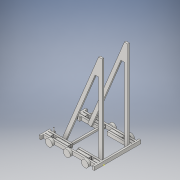
# Autodesk Inventor part: base
Saved by Autodesk Inventor 2016 (Build 200138000, 138)
## iProperties
Created: 2018-01-19
Part Number: base
Material: Generic
Document SubType Name: Modeling
Designer: New User
Density: 1 g/cm^3
Appearance: Default
Author: New User
Autodesk Inventor part; units mm, degrees
ref_plane "YZ Plane" through (0, 0, 0) normal (1, 0, 0) x (0, 1, 0)
ref_plane "XZ Plane" through (0, 0, 0) normal (0, 1, 0) x (-1, 0, 0)
ref_plane "XY Plane" through (0, 0, 0) normal (0, 0, 1) x (1, 0, 0)
sketch "Sketch1" plane through (0, 0, 0) normal (0, 1, 0) x (-1, 0, 0)
  line L0 (0, -685.8) -> (0, 0)
  line L1 (25.4, -38.1) -> (689.3542, -38.1)
  line L2 (787.4, -63.5) -> (25.4, -63.5)
  line L3 (787.4, -647.7) -> (25.4, -647.7)
  line L4 (787.4, -622.3) -> (25.4, -622.3)
  line L5 (787.4, -114.3) -> (457.2, -114.3)
  line L6 (457.2, -114.3) -> (457.2, -139.7)
  line L7 (457.2, -546.1) -> (457.2, -571.5)
  line L8 (457.2, -571.5) -> (787.4, -571.5)
  line L9 (25.4, -571.5) -> (355.6, -571.5)
  line L10 (355.6, -571.5) -> (355.6, -546.1)
  line L11 (355.6, -546.1) -> (25.4, -546.1)
  line L12 (25.4, -139.7) -> (355.6, -139.7)
  line L13 (355.6, -114.3) -> (25.4, -114.3)
  line L14 (355.6, -114.3) -> (355.6, -139.7)
  line L15 (0, 0) -> (25.4, 0)
  line L16 (787.4, 0) -> (812.8, 0)
  line L17 (787.4, -63.5) -> (787.4, -114.3)
  line L18 (787.4, -571.5) -> (787.4, -622.3)
  line L19 (787.4, -647.7) -> (787.4, -685.8)
  line L20 (812.8, -685.8) -> (787.4, -685.8)
  line L21 (25.4, -685.8) -> (0, -685.8)
  line L22 (25.4, -647.7) -> (25.4, -685.8)
  line L23 (25.4, -571.5) -> (25.4, -622.3)
  line L24 (25.4, -139.7) -> (25.4, -546.1)
  line L25 (25.4, 0) -> (25.4, -38.1)
  line L26 (25.4, -63.5) -> (25.4, -114.3)
  line L27 (689.3542, -38.1) -> (787.4, -38.1)
  line L28 (787.4, -38.1) -> (787.4, 0)
  line L29 (812.8, -152.4) -> (787.4, -152.4)
  line L30 (787.4, -533.4) -> (812.8, -533.4)
  line L31 (812.8, 0) -> (812.8, -152.4)
  line L32 (812.8, -533.4) -> (812.8, -685.8)
  line L33 (787.4, -139.7) -> (787.4, -152.4)
  line L34 (508, -139.7) -> (508, -546.1)
  line L35 (482.6, -139.7) -> (482.6, -546.1)
  line L36 (457.2, -139.7) -> (482.6, -139.7)
  line L37 (508, -139.7) -> (787.4, -139.7)
  line L38 (660.4, -546.1) -> (508, -546.1)
  line L39 (482.6, -546.1) -> (457.2, -546.1)
  line L40 (660.4, -546.1) -> (787.4, -546.1)
  line L41 (787.4, -546.1) -> (787.4, -533.4)
  dimension "d0" = 685.8
  dimension "d1" = 812.8
  dimension "d4" = 25.4
  dimension "d5" = 25.4
  dimension "d8" = 50.8
  dimension "d9" = 25.4
  dimension "d10" = 50.8
  dimension "d42" = 330.2
  dimension "d43" = 25.4
  dimension "d44" = 25.4
  dimension "d45" = 25.4
  dimension "d46" = 25.4
  dimension "d47" = 330.2
  dimension "d54" = 152.4
  dimension "d55" = 152.4
  dimension "d56" = 25.4
  dimension "d57" = 304.8
  constraints: 84 end point, 74 perpendicular, 7 horizontal, 6 parallel, 4 point on line, 3 equal length
  measures "d0" distance of L16.end L20.start
  measures "d1" distance of L20.start L0.start
  measures "d4" distance between parallel lines of L3 L4
  measures "d5" distance between parallel lines of L2 L1
  measures "d8" distance between parallel lines of L4 L9
  measures "d9" distance of L9.end L10.end
  measures "d10" distance between parallel lines of L2 L5
  measures "d42" distance between parallel lines of L10 L23
  measures "d43" distance between parallel lines of L23 L0
  measures "d44" distance between parallel lines of L0 L24
  measures "d45" distance between parallel lines of L0 L26
  measures "d46" distance between parallel lines of L0 L25
  measures "d47" distance of L7.end L8.end
  measures "d54" distance between parallel lines of L20 L30
  measures "d55" distance between parallel lines of L16 L29
  measures "d56" distance between parallel lines of L35 L34
  measures "d57" distance between parallel lines of L34 L31
extrude "Extrusion1" add sketch "Sketch1" along normal blind 50.8
sketch "Sketch2" plane through (-689.3542, 0, -38.1) normal (0, 0, 1) x (1, 0, 0)
  circle A0 centre (16.2542, 17.78) radius 50.8
  circle A1 centre (282.9542, 17.78) radius 50.8
  circle A2 centre (549.6542, 17.78) radius 50.8
  line L0 (-98.0458, 0) -> (-98.0458, 50.8) projected
  line L1 (663.9542, 0) -> (663.9542, 50.8) projected
  line L2 (-98.0458, 0) -> (663.9542, 0) projected
  point P0 (689.3542, 0)
  dimension "d13" = 101.6
  dimension "d14" = 114.3
  dimension "d15" = 114.3
  dimension "d16" = 381
  dimension "d17" = 17.78
  dimension "d18" = 17.78
  dimension "d19" = 17.78
  constraints: 3 centre point, 2 equal radius
  measures "d13" diameter of A0
  measures "d14" distance from line of L0 A0.centre
  measures "d15" distance from line of L1 A2.centre
  measures "d16" distance from line of L0 A1.centre
  measures "d17" distance from line of L2 A0.centre
  measures "d18" distance from line of L2 A1.centre
  measures "d19" distance from line of L2 A2.centre
extrude "Extrusion2" add sketch "Sketch2" along normal blind 38.1
sketch "Sketch3" plane through (-25.4, 0, -647.7) normal (0, 0, -1) x (-1, 0, 0)
  arc A0 (152.9047, 50.8) -> (75.6953, 50.8) centre (114.3, 17.78) ccw projected
  circle A1 centre (114.3, 17.78) radius 50.8
  arc A2 (419.6047, 50.8) -> (342.3953, 50.8) centre (381, 17.78) ccw projected
  circle A3 centre (381, 17.78) radius 50.8
  arc A4 (686.3047, 50.8) -> (609.0953, 50.8) centre (647.7, 17.78) ccw projected
  circle A5 centre (647.7, 17.78) radius 50.8
  point P0 (-25.4, 0)
  constraints: 3 centre point, 3 coincident
extrude "Extrusion3" add sketch "Sketch3" along normal blind 38.1
sketch "Sketch4" plane through (-25.4, 0, -63.5) normal (-1, 0, 0) x (0, 0, 1)
  line L0 (-50.8, 50.8) -> (0, 50.8) projected
  line L1 (0, 0) -> (-50.8, 0) projected
  line L2 (-6.35, 50.8) -> (-44.45, 50.8)
  line L3 (-50.8, 44.45) -> (-50.8, 6.35)
  line L4 (-44.45, 0) -> (-6.35, 0)
  line L5 (0, 6.35) -> (0, 44.45)
  arc A0 (-44.45, 50.8) -> (-50.8, 44.45) centre (-44.45, 44.45) ccw
  arc A1 (-50.8, 6.35) -> (-44.45, 0) centre (-44.45, 6.35) ccw
  arc A2 (0, 44.45) -> (-6.35, 50.8) centre (-6.35, 44.45) ccw
  arc A3 (-6.35, 0) -> (0, 6.35) centre (-6.35, 6.35) ccw
  line L6 (-558.8, 50.8) -> (-508, 50.8) projected
  line L7 (-508, 0) -> (-508, 50.8) projected
  line L8 (-552.45, 50.8) -> (-514.35, 50.8)
  line L9 (-508, 44.45) -> (-508, 6.35)
  line L10 (-514.35, 0) -> (-552.45, 0)
  line L11 (-558.8, 6.35) -> (-558.8, 44.45)
  arc A4 (-508, 44.45) -> (-514.35, 50.8) centre (-514.35, 44.45) ccw
  arc A5 (-558.8, 6.35) -> (-552.45, 0) centre (-552.45, 6.35) ccw
  arc A6 (-552.45, 50.8) -> (-558.8, 44.45) centre (-552.45, 44.45) ccw
  arc A7 (-514.35, 0) -> (-508, 6.35) centre (-514.35, 6.35) ccw
  line L12 (-552.45, 3.175) -> (-514.35, 3.175)
  arc A8 (-514.35, 3.175) -> (-511.175, 6.35) centre (-514.35, 6.35) ccw
  line L13 (-511.175, 6.35) -> (-511.175, 44.45)
  arc A9 (-511.175, 44.45) -> (-514.35, 47.625) centre (-514.35, 44.45) ccw
  line L14 (-514.35, 47.625) -> (-552.45, 47.625)
  arc A10 (-552.45, 47.625) -> (-555.625, 44.45) centre (-552.45, 44.45) ccw
  line L15 (-555.625, 44.45) -> (-555.625, 6.35)
  arc A11 (-555.625, 6.35) -> (-552.45, 3.175) centre (-552.45, 6.35) ccw
  line L16 (-6.35, 3.175) -> (-44.45, 3.175)
  arc A12 (-47.625, 6.35) -> (-44.45, 3.175) centre (-44.45, 6.35) ccw
  line L17 (-47.625, 6.35) -> (-47.625, 44.45)
  arc A13 (-44.45, 47.625) -> (-47.625, 44.45) centre (-44.45, 44.45) ccw
  line L18 (-44.45, 47.625) -> (-6.35, 47.625)
  arc A14 (-3.175, 44.45) -> (-6.35, 47.625) centre (-6.35, 44.45) ccw
  line L19 (-3.175, 44.45) -> (-3.175, 6.35)
  arc A15 (-6.35, 3.175) -> (-3.175, 6.35) centre (-6.35, 6.35) ccw
  point P0 (63.5, 0)
  dimension "d24" = 6.35
  dimension "d25" = 6.35
  constraints: 32 end point, 32 point on circle, 16 centre point, 16 tangent, 8 parallel, 8 point on line, 6 equal radius, 4 perpendicular, 2 horizontal, 14 other
  measures "d24" radius of A0
  measures "d25" radius of A4
extrude "Extrusion4" add sketch "Sketch4" along normal blind 762 contours L0 A2 L5 A3 L1 A1 L3 A0 | L6 A4 L7 A7 L10 A5 L11 A6
sketch "Sketch5" plane through (0, 50.8, 0) normal (0, 1, 0) x (1, 0, 0)
  line L0 (-25.4, 63.5) -> (-787.4, 63.5) projected
  line L1 (-355.6, 114.3) -> (-25.4, 114.3) projected
  line L2 (-101.6, 63.5) -> (-152.4, 63.5)
  line L3 (-152.4, 63.5) -> (-152.4, 114.3)
  line L4 (-152.4, 114.3) -> (-101.6, 114.3)
  line L5 (-101.6, 114.3) -> (-101.6, 63.5)
  line L6 (-355.6, 114.3) -> (-457.2, 114.3) projected
  line L7 (-342.9, 63.5) -> (-457.2, 63.5)
  line L8 (-457.2, 63.5) -> (-457.2, 114.3)
  line L9 (-457.2, 114.3) -> (-342.9, 114.3)
  line L10 (-342.9, 114.3) -> (-342.9, 63.5)
  line L11 (-787.4, 114.3) -> (-457.2, 114.3) projected
  line L12 (-647.7, 63.5) -> (-711.2, 63.5)
  line L13 (-711.2, 63.5) -> (-711.2, 114.3)
  line L14 (-711.2, 114.3) -> (-647.7, 114.3)
  line L15 (-647.7, 114.3) -> (-647.7, 63.5)
  line L16 (-457.2, 571.5) -> (-787.4, 571.5) projected
  line L17 (-25.4, 622.3) -> (-787.4, 622.3) projected
  line L18 (-711.2, 571.5) -> (-647.7, 571.5)
  line L19 (-647.7, 571.5) -> (-647.7, 622.3)
  line L20 (-647.7, 622.3) -> (-711.2, 622.3)
  line L21 (-711.2, 622.3) -> (-711.2, 571.5)
  line L22 (-355.6, 571.5) -> (-457.2, 571.5) projected
  line L23 (-457.2, 571.5) -> (-355.6, 571.5)
  line L24 (-355.6, 571.5) -> (-355.6, 622.3)
  line L25 (-355.6, 622.3) -> (-457.2, 622.3)
  line L26 (-457.2, 622.3) -> (-457.2, 571.5)
  line L27 (-25.4, 571.5) -> (-355.6, 571.5) projected
  line L28 (-165.1, 622.3) -> (-101.6, 622.3)
  line L29 (-101.6, 622.3) -> (-101.6, 571.5)
  line L30 (-101.6, 571.5) -> (-165.1, 571.5)
  line L31 (-165.1, 571.5) -> (-165.1, 622.3)
  line L32 (-25.4, 546.1) -> (-25.4, 139.7) projected
  line L33 (-787.4, 139.7) -> (-787.4, 152.4) projected
  point P0 (0, 0)
  point P1 (-787.4, 546.1)
  dimension "d28" = 63.5
  dimension "d29" = 50.8
  dimension "d30" = 76.2
  dimension "d31" = 76.2
  dimension "d32" = 63.5
  dimension "d33" = 63.5
  dimension "d34" = 76.2
  dimension "d35" = 190.5
  dimension "d36" = 190.5
  dimension "d37" = 190.5
  dimension "d38" = 190.5
  constraints: 48 end point, 13 point on line, 12 parallel, 6 horizontal, 6 perpendicular
  measures "d28" distance of L29.end L30.end
  measures "d29" distance of L3.end L4.end
  measures "d30" distance between parallel lines of L32 L29
  measures "d31" distance between parallel lines of L32 L5
  measures "d32" distance between parallel lines of L21 L19
  measures "d33" distance between parallel lines of L13 L15
  measures "d34" distance between parallel lines of L33 L21
  measures "d35" distance between parallel lines of L19 L26
  measures "d36" distance between parallel lines of L8 L15
  measures "d37" distance between parallel lines of L24 L31
  measures "d38" distance between parallel lines of L10 L3
extrude "Extrusion5" cut sketch "Sketch5" against normal blind 50.8 contours L0 L3 L1 L5 | L0 L8 L6 L1 L10 | L0 L13 L11 L15 | L26 L17 L24 L22 | L16 L21 L17 L19 | L31 L17 L29 L27
sketch "Sketch7" plane through (-25.4, 0, -139.7) normal (0, 0, -1) x (-1, 0, 0)
  point P0 (-25.4, 0)
sketch "Sketch8" plane through (0, 50.8, 0) normal (0, 1, 0) x (1, 0, 0)
  line L0 (-508, 139.7) -> (-787.4, 139.7) projected
  line L1 (-508, 139.7) -> (-482.6, 139.7)
  line L2 (-482.6, 139.7) -> (-482.6, 546.1)
  line L3 (-482.6, 546.1) -> (-508, 546.1)
  line L4 (-508, 546.1) -> (-508, 139.7)
  point P0 (0, 0)
  constraints: 8 end point, 2 parallel, 1 horizontal, 1 perpendicular
extrude "Extrusion7" cut sketch "Sketch8" against normal blind 25.4
sketch "Sketch9" plane through (-25.4, 0, -139.7) normal (0, 0, -1) x (-1, 0, 0)
  line L0 (330.2, 0) -> (0, 0) projected
  line L1 (0, 0) -> (50.8, 0)
  line L2 (50.8, 0) -> (50.8, 993.775)
  line L3 (50.8, 1346.2) -> (0, 1346.2)
  line L4 (0, 1346.2) -> (0, 0)
  line L5 (609.0953, 50.8) -> (419.6047, 50.8) projected
  line L6 (50.8, 1346.2) -> (584.2, 50.8)
  line L7 (584.2, 50.8) -> (537.2264, 31.4579)
  line L8 (537.2264, 31.4579) -> (101.7518, 1089.0389)
  line L9 (50.8, 1089.0389) -> (101.7518, 1089.0389)
  line L10 (50.8, 993.775) -> (50.8, 1089.0389)
  point P0 (-25.4, 0)
  dimension "d61" = 1346.2
  dimension "d67" = 50.8
  dimension "d68" = 50.8
  constraints: 18 end point, 3 parallel, 3 perpendicular, 2 horizontal, 1 point on line
  measures "d61" distance of L3.end L0.end
  measures "d67" distance between parallel lines of L6 L8
  measures "d68" distance between parallel lines of L4 L2
extrude "Extrusion8" add sketch "Sketch9" along normal blind 25.4
sketch "Sketch10" plane through (-355.6, 0, -546.1) normal (0, 0, 1) x (1, 0, 0)
  line L0 (-431.8, 0) -> (330.2, 0) projected
  line L1 (330.2, 0) -> (279.4, 0)
  line L2 (279.4, 1346.2) -> (330.2, 1346.2)
  line L3 (330.2, 1346.2) -> (330.2, 0)
  line L4 (279.4, 1346.2) -> (-260.35, 31.75)
  line L5 (-260.35, 31.75) -> (-213.3576, 12.4536)
  line L6 (-213.3576, 12.4536) -> (166.1331, 936.625)
  line L7 (279.4, 909.6375) -> (279.4, 0)
  line L8 (330.2, 50.8) -> (254.5047, 50.8) projected
  line L9 (279.4, 1089.0389) -> (228.7185, 1089.0389)
  line L10 (166.1331, 936.625) -> (228.7185, 1089.0389)
  line L11 (279.4, 909.6375) -> (279.4, 1089.0389)
  line L12 (279.4, 50.8) -> (279.4, 1089.0389) projected
  point P0 (355.6, 0)
  point P1 (279.4, 1212.7791)
  constraints: 20 end point, 2 horizontal, 2 parallel, 1 collinear, 1 perpendicular, 1 vertical
extrude "Extrusion9" add sketch "Sketch10" along normal blind 25.4
sketch "Sketch11" plane through (-787.4, 0, -546.1) normal (0, 0, 1) x (1, 0, 0)
  line L0 (25.4, 0) -> (50.8, 0)
  line L1 (50.8, 0) -> (50.8, 50.8)
  line L2 (50.8, 50.8) -> (25.4, 50.8)
  line L3 (25.4, 50.8) -> (25.4, 0)
  line L4 (0, 0) -> (0, 50.8) projected
  point P0 (787.4, 0)
  dimension "d75" = 25.4
  dimension "d76" = 50.8
  dimension "d77" = 25.4
  constraints: 8 end point, 2 parallel, 1 horizontal, 1 perpendicular
  measures "d75" distance of L1.end L2.end
  measures "d76" distance of L2.end L0.start
  measures "d77" distance between parallel lines of L3 L4
extrude "Extrusion10" add sketch "Sketch11" along normal blind 25.4
sketch "Sketch12" plane through (-508, 0, -139.7) normal (0, 0, -1) x (-1, 0, 0)
  line L0 (203.2, 0) -> (279.4, 0) projected
  line L1 (254, 0) -> (228.6, 0)
  line L2 (228.6, 0) -> (228.6, 50.8)
  line L3 (228.6, 50.8) -> (254, 50.8)
  line L4 (254, 50.8) -> (254, 0)
  line L5 (279.4, 0) -> (279.4, 50.8) projected
  point P0 (-508, 0)
  dimension "d80" = 25.4
  dimension "d81" = 25.4
  constraints: 8 end point, 2 parallel, 1 horizontal, 1 perpendicular, 1 point on line
  measures "d80" distance of L2.end L3.end
  measures "d81" distance between parallel lines of L5 L4
extrude "Extrusion11" add sketch "Sketch12" along normal blind 25.4
sketch "Sketch13" plane through (0, 50.8, 0) normal (0, 1, 0) x (1, 0, 0)
  circle A0 centre (-749.3, 533.4) radius 6.35
  circle A1 centre (-749.3, 152.4) radius 6.35
  line L0 (-736.6, 520.7) -> (-762, 520.7) projected
  line L1 (-736.6, 546.1) -> (-736.6, 520.7) projected
  line L2 (-736.6, 139.7) -> (-736.6, 165.1) projected
  line L3 (-736.6, 165.1) -> (-762, 165.1) projected
  point P0 (0, 0)
  dimension "d84" = 12.7
  dimension "d85" = 12.7
  dimension "d86" = 12.7
  dimension "d87" = 12.7
  dimension "d88" = 12.7
  dimension "d89" = 12.7
  constraints: 2 centre point
  measures "d84" diameter of A0
  measures "d85" distance from line of L0 A0.centre
  measures "d86" distance from line of L1 A0.centre
  measures "d87" diameter of A1
  measures "d88" distance from line of L2 A1.centre
  measures "d89" distance from line of L3 A1.centre
extrude "Extrusion12" add sketch "Sketch13" along normal blind 50.8
body "Solid1"
